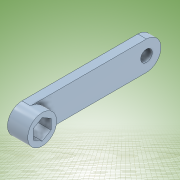
# Autodesk Inventor part: Transmision_Inf
Saved by Autodesk Inventor 2022 (Build 260153000, 153)
## iProperties
Created: 2022-02-14
Part Number: Transmision_Inf
Material: Genérico
Document SubType Name: Modeling
Designer: Marco
Density: 1 g/cm^3
Appearance: Azul acero
Author: Marco
Autodesk Inventor part; units mm, degrees
ref_plane "YZ Plane" through (0, 0, 0) normal (1, 0, 0) x (0, 1, 0)
ref_plane "XZ Plane" through (0, 0, 0) normal (0, 1, 0) x (-1, 0, 0)
ref_plane "XY Plane" through (0, 0, 0) normal (0, 0, 1) x (1, 0, 0)
sketch "Boceto1" plane through (0, 0, 0) normal (1, 0, 0) x (0, 1, 0)
  arc A0 (5, 0) -> (-5, 0) centre (0, 0) ccw
  arc A1 (-5, -40) -> (5, -40) centre (0, -40) ccw
  line L0 (5, 0) -> (5, -40)
  line L1 (-5, -40) -> (-5, 0)
  circle A2 centre (0, -40) radius 2
  dimension "d1" = 10
  dimension "d2" = 10
  dimension "d3" = 40
  dimension "d4" = 4
  constraints: 6 point on circle, 4 end point, 3 centre point, 3 coincident, 3 horizontal alignment, 2 point on line, 1 tangent, 1 vertical alignment
  measures "d1" diameter of A0
  measures "d2" diameter of A1
  measures "d3" distance of A1.centre point (0, 0)
  measures "d4" diameter of A2
extrude "Extrusión1" add sketch "Boceto1" along normal blind 3
sketch "Boceto2" plane through (3, 0, 0) normal (1, 0, 0) x (0, 0, -1)
  circle A0 centre (0, 0) radius 5
  constraints: 1 centre point, 1 coincident
extrude "Extrusión2" add sketch "Boceto2" along normal blind 4
sketch "Boceto3" plane through (7, 0, 0) normal (1, 0, 0) x (0, 0, -1)
  line L0 (0, 3.5218) -> (3.05, 1.7609)
  line L1 (3.05, 1.7609) -> (3.05, -1.7609)
  line L2 (3.05, -1.7609) -> (0, -3.5218)
  line L3 (0, -3.5218) -> (-3.05, -1.7609)
  line L4 (-3.05, -1.7609) -> (-3.05, 1.7609)
  line L5 (-3.05, 1.7609) -> (0, 3.5218)
  point P0 (0, 0)
  point P1 (0, 0)
  point P2 (3.05, 0)
  dimension "d10" = 6.1
  constraints: 12 end point, 1 coincident, 1 horizontal alignment, 1 midpoint, 13 other
  measures "d10" distance of L1.end L3.end
extrude "Extrusión3" cut sketch "Boceto3" against normal blind 6.8
